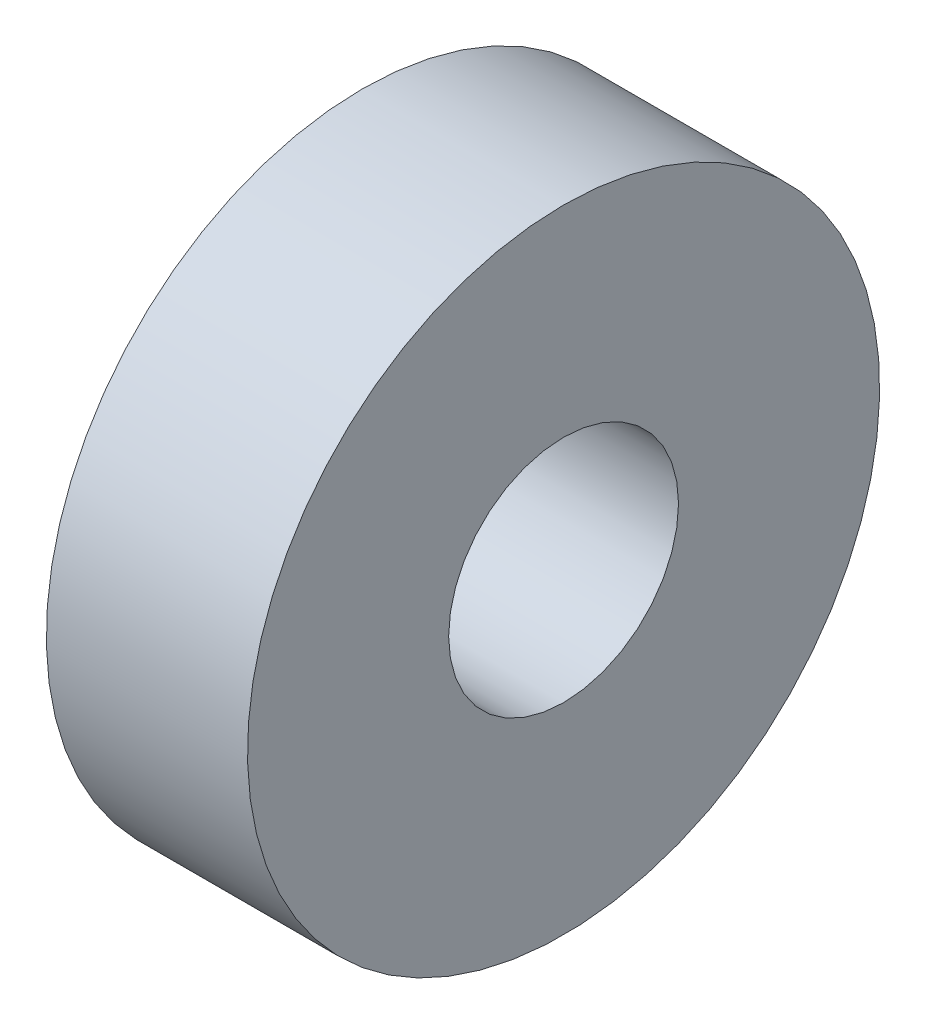
# Autodesk Inventor part: bearing
Saved by Autodesk Inventor 2023 (Build 270158000, 158)
## iProperties
Created: 2023-02-17
Part Number: bearing
Material: Generic
Document SubType Name: Modeling
Designer: shrey
Density: 1 g/cm^3
Appearance: Gunmetal - Polished
Author: shrey
Autodesk Inventor part; units mm, degrees
ref_plane "YZ Plane" through (0, 0, 0) normal (1, 0, 0) x (0, 1, 0)
ref_plane "XZ Plane" through (0, 0, 0) normal (0, 1, 0) x (-1, 0, 0)
ref_plane "XY Plane" through (0, 0, 0) normal (0, 0, 1) x (1, 0, 0)
ref_plane "Work Plane1" through (-3, -630, 117.5) normal (-1, 0, 0) x (0, 1, 0)
sketch "Sketch1" plane through (-3, -630, 117.5) normal (-1, 0, 0) x (0, 1, 0)
  line L0 (19.7, -17.2) -> (19.7, 17.2) projected
  line L1 (19.7, 17.2) -> (-19.7, 17.2) projected
  line L2 (-19.7, 17.2) -> (-19.7, -17.2) projected
  line L3 (-19.7, -17.2) -> (19.7, -17.2) projected
  circle A0 centre (2.5, 0) radius 4 projected
  circle A1 centre (2.5, 0) radius 4
  circle A2 centre (2.5, 0) radius 11
  point P0 (630, 117.5)
  dimension "d0" = 8
  dimension "d1" = 22
  constraints: 2 centre point, 2 coincident
  measures "d0" diameter of A1
  measures "d1" diameter of A2
extrude "Extrusion1" add sketch "Sketch1" along normal blind 7 contours A2
body "Solid1"
